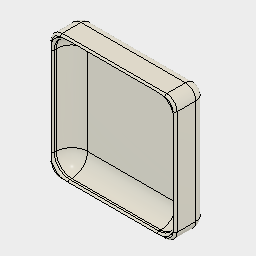
tray (Autodesk Fusion 360 design; units mm, degrees)
Autodesk Fusion 360 part; units mm, degrees
note: some values were not read from the file. Set by a fixed rule: which face or edge a step refers to.
sketch "Sketch1" plane through (0, 0, 0) normal (1, 0, 0) x (0, 0, -1)
sketch "Sketch2" plane through (0, 0, 0) normal (0, 0, 1) x (1, 0, 0)
  line L0 (30, -30) -> (-30, -30)
  line L1 (-30, -30) -> (-30, 30)
  line L2 (-30, 30) -> (30, 30)
  line L3 (30, 30) -> (30, -30)
  line L4 (30, -30) -> (-30, 30) construction
  line L5 (-30, -30) -> (30, 30) construction
  dimension "d1" = 60
  dimension "d2" = 60
  measures "d1" distance of L1.end L2.end
  measures "d2" distance of L0.end L1.end
extrude "Extrude1" add sketch "Sketch2" along normal blind 15
shell "Shell1" thickness 1.2 removed faces 1 at (10, -10, 15)
extrude "Extrude2" add 1 faces at (9.6, -9.6, 1.2) along direction (0, 0, 1) blind 4.4
sketch "Sketch3" plane through (0, 0, 0) normal (0, 0, -1) x (-1, 0, 0)
  line L0 (30, 30) -> (-30, 30)
  line L1 (-30, 30) -> (-30, -30)
  line L2 (-30, -30) -> (30, -30)
  line L3 (30, -30) -> (30, 30)
  line L4 (-28.8, 28.8) -> (28.8, 28.8)
  line L5 (28.8, 28.8) -> (28.8, -28.8)
  line L6 (28.8, -28.8) -> (-28.8, -28.8)
  line L7 (-28.8, -28.8) -> (-28.8, 28.8)
  line L8 (-28.8, -28.8) -> (28.8, 28.8) construction
  line L9 (-28.8, 28.8) -> (28.8, -28.8) construction
  circle A0 centre (17.5, -17.5) radius 2.5
  line L10 (-1.75, 0) -> (-22.5, 0)
  line L11 (0, 1.75) -> (0, 22.5)
  circle A1 centre (-17.5, -17.5) radius 2.5
  circle A2 centre (-17.5, 17.5) radius 2.5
  circle A3 centre (17.5, 17.5) radius 2.5
  line L12 (17.5, -17.5) -> (-17.5, -17.5) construction
  line L13 (-17.5, -17.5) -> (-17.5, 17.5) construction
  line L14 (-17.5, 17.5) -> (17.5, 17.5) construction
  line L15 (17.5, 17.5) -> (17.5, -17.5) construction
  line L16 (17.5, -17.5) -> (-17.5, 17.5) construction
  line L17 (-17.5, -17.5) -> (17.5, 17.5) construction
  circle A4 centre (0, 0) radius 2.5
  dimension "d8" = 5
  dimension "d9" = 5
  dimension "d10" = 5
  dimension "d13" = 35
  dimension "d14" = 5
  dimension "d22" = 5
  measures "d8" diameter of A0
  measures "d9" diameter of A1
  measures "d10" diameter of A3
  measures "d13" distance of A2.centre A3.centre
  measures "d14" diameter of A4
  measures "d22" diameter of A2
extrude "Extrude3" cut sketch "Sketch3" against normal blind 5 contours A0 | A1 | A2 | A3 | A4
fillet "Fillet1" radius 7.5 8 edges at (28.8, -28.8, 10.3) (0, -28.8, 5.6) (28.8, 0, 5.6) (0, 28.8, 5.6) (28.8, 28.8, 10.3) (-28.8, 28.8, 10.3) (-28.8, 0, 5.6) (-28.8, -28.8, 10.3)
fillet "Fillet2" radius 5 8 edges at (30, 30, 7.5) (-30, 30, 7.5) (0, 30, 0) (30, 0, 0) (30, -30, 7.5) (-30, 0, 0) (-30, -30, 7.5) (0, -30, 0)
chamfer "Chamfer1" distance 1 angle 45 5 edges at (-15.1692, -16.596, 0) (19.8308, -16.596, 0) (19.8308, 18.404, 0) (-15.1692, 18.404, 0) (2.3308, 0.904, 0)
fillet "Fillet3" radius 1 16 edges at (-26.6033, -26.6033, 15) (-28.8, 0, 15) (-26.6033, 26.6033, 15) (0, 28.8, 15) (26.6033, 26.6033, 15) (28.8, 0, 15) (26.6033, -26.6033, 15) (0, -28.8, 15) (-28.5355, 28.5355, 15) (-30, 0, 15) (-28.5355, -28.5355, 15) (0, -30, 15) (28.5355, -28.5355, 15) (30, 0, 15) (28.5355, 28.5355, 15) (0, 30, 15)
equation "d6 = 5.6 mm - 1.2 mm"
equation "d9 = d8"
equation "d10 = d8"
equation "d14 = d10"
equation "d22 = d9"
